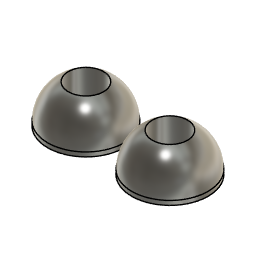
brake line end conector v2 (Autodesk Fusion 360 design; units mm, degrees)
Autodesk Fusion 360 part; units mm, degrees
sketch "Sketch1" plane through (0, 0, 0) normal (0, 0, 1) x (1, 0, 0)
  circle A0 centre (7.168, 10.1087) radius 1.15
  circle A1 centre (7.168, 10.1087) radius 2.5
  dimension "d1" = 2.3
  dimension "d3" = 5
  measures "d1" diameter of A0
  measures "d3" diameter of A1
extrude "Extrude1" add sketch "Sketch1" along normal blind 2.5 makes body 1
fillet "Fillet1" radius 2.5 1 edges at (4.8372, 9.2047, 2.5) on bodies 1
copy_body "CopyPasteBodies1" bodies 1 makes body 2
move_body "Move1" bodies 2 to x (1, 0, 0) y (0, 1, 0) z (0, 0, 1) at (5.5, 0, 0)
